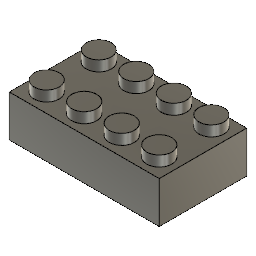
lego box 2 (v2~recovered) (Autodesk Fusion 360 design; units mm, degrees)
Autodesk Fusion 360 part; units mm, degrees
box "BoxPrimitive1" add length 42 width 72 height 20 placed x (0, 1, 0) y (-1, 0, 0) z (0, 0, 1) at (72, 0, 0)
sketch "Sketch2" plane through (0, 0, 20) normal (0, 0, 1) x (-1, 0, 0)
  line L0 (-72, -42) -> (0, -42)
  line L1 (0, -42) -> (0, 0)
  line L2 (0, 0) -> (-72, 0)
  line L3 (-72, 0) -> (-72, -42)
  circle A0 centre (-9, -9) radius 6
  circle A1 centre (-9, -34) radius 6
  circle A2 centre (-27, -34) radius 6
  circle A3 centre (-45, -34) radius 6
  circle A4 centre (-63, -34) radius 6
  circle A5 centre (-27, -9) radius 6
  circle A6 centre (-45, -9) radius 6
  circle A7 centre (-63, -9) radius 6
  point P0 (-27, -9)
  point P1 (-45, -9)
  point P2 (-63, -9)
  point P3 (-9, -34)
  point P4 (-27, -34)
  point P5 (-45, -34)
  point P6 (-63, -34)
  dimension "d6" = 12
  dimension "d9" = 54
  dimension "d10" = 25
  dimension "d11" = 12
  dimension "d12" = 12
  dimension "d13" = 12
  dimension "d14" = 12
  dimension "d15" = 12
  dimension "d16" = 12
  dimension "d17" = 12
  constraint coincident P3 A1.centre
  constraint coincident P4 A2.centre
  constraint coincident P5 A3.centre
  constraint coincident P6 A4.centre
  constraint coincident P0 A5.centre
  constraint coincident P1 A6.centre
  constraint coincident P2 A7.centre
  measures "d6" diameter of A0
  measures "d11" diameter of A1
  measures "d12" diameter of A2
  measures "d13" diameter of A3
  measures "d14" diameter of A4
  measures "d15" diameter of A5
  measures "d16" diameter of A6
  measures "d17" diameter of A7
sketch "Sketch3" plane through (0, 0, 20) normal (0, 0, 1) x (1, 0, 0)
sketch "Sketch4" plane through (0, 0, 20) normal (0, 0, 1) x (1, 0, 0)
extrude "Extrude1" add sketch "Sketch2" along normal blind 5 contours A0 | A1 | A2 | A3 | A4 | A5 | A6 | A7
shell "Shell1" thickness 2.5 removed faces 1 at (24, 14, 0)
